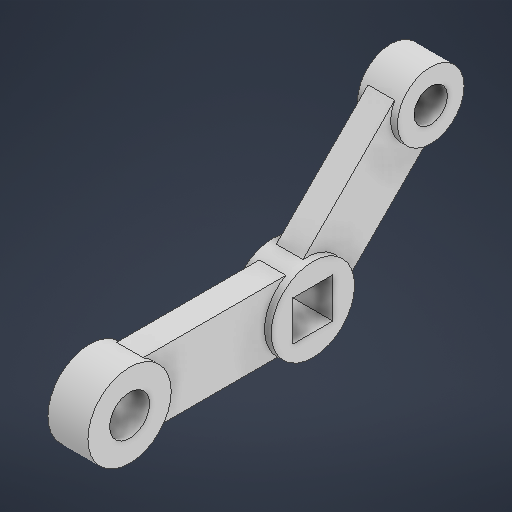
# Autodesk Inventor part: Part4
Saved by Autodesk Inventor 2026 (Build 300175050, 175E)
## iProperties
Created: 2026-04-09
Part Number: Part4
Material: Generic
Document SubType Name: Modeling
Designer: Administrator
Density: 1 g/cm^3
Appearance: Default
Author: Administrator
Autodesk Inventor part; units mm, degrees
ref_plane "YZ Plane" through (0, 0, 0) normal (1, 0, 0) x (0, 1, 0)
ref_plane "XZ Plane" through (0, 0, 0) normal (0, 1, 0) x (-1, 0, 0)
ref_plane "XY Plane" through (0, 0, 0) normal (0, 0, 1) x (1, 0, 0)
sketch "Sketch1" plane through (0, 0, 0) normal (1, 0, 0) x (0, 1, 0)
  circle A0 centre (0, 0) radius 12.5
  line L0 (0, 0) -> (0, -55) construction
  circle A1 centre (0, -55) radius 12.5
  line L1 (0, -55) -> (35.3553, -90.3553) construction
  circle A2 centre (35.3553, -90.3553) radius 10
  line L2 (10.9114, -6.0985) -> (10.9114, -48.9015)
  line L3 (-9.0886, -8.5818) -> (-9.0886, -46.4182)
  line L4 (40.0876, -81.5459) -> (12.4612, -54.0158)
  line L5 (0.7049, -67.4801) -> (25.5516, -92.3268)
  dimension "d0" = 25
  dimension "d1" = 55
  dimension "d2" = 25
  dimension "d3" = 50
  dimension "d4" = 20
  dimension "d5" = 20
  dimension "d7" = 45
  dimension "d8" = 0.1
  constraints: 12 end point, 8 point on circle, 3 centre point, 3 coincident, 3 vertical, 1 parallel
  measures "d0" diameter of A0
  measures "d1" distance of L0.start L0.end
  measures "d2" diameter of A1
  measures "d3" distance of L1.start L1.end
  measures "d4" diameter of A2
  measures "d5" distance between parallel lines of L3 L2
  measures "d7" angle of L1 L0
  measures "d8" angle of L5 L4
extrude "Extrusion1" add sketch "Sketch1" along normal mid plane 8
sketch "Sketch2" plane through (4, 0, 0) normal (1, 0, 0) x (0, 0, -1)
  circle A0 centre (0, 0) radius 12.5
  line L0 (0, 0) -> (55, 0) construction
  circle A1 centre (55, 0) radius 12.5
  line L1 (55, 0) -> (90.3553, 35.3553)
  circle A2 centre (90.3553, 35.3553) radius 10
  dimension "d11" = 25
  dimension "d12" = 55
  dimension "d13" = 25
  dimension "d14" = 50
  dimension "d15" = 45
  dimension "d16" = 20
  constraints: 4 end point, 3 centre point, 3 coincident, 1 horizontal
  measures "d11" diameter of A0
  measures "d12" distance of L0.start L0.end
  measures "d13" diameter of A1
  measures "d14" distance of L1.start L1.end
  measures "d15" angle of L0 L1
  measures "d16" diameter of A2
extrude "Extrusion2" add sketch "Sketch2" along normal blind 2
sketch "Sketch3" plane through (-4, 0, 0) normal (-1, 0, 0) x (0, 0, 1)
  line L0 (0, 0) -> (-55, 0) construction
  line L1 (-55, 0) -> (-90.3553, 35.3553) construction
  circle A0 centre (-90.3553, 35.3553) radius 10
  circle A1 centre (-55, 0) radius 12.5
  circle A2 centre (0, 0) radius 12.5
  dimension "d19" = 55
  dimension "d20" = 50
  dimension "d21" = 45
  dimension "d22" = 20
  dimension "d23" = 25
  dimension "d24" = 25
  constraints: 4 end point, 3 centre point, 3 coincident, 1 horizontal
  measures "d19" distance of L0.start L0.end
  measures "d20" distance of L0.end L1.end
  measures "d21" angle of L0 L1
  measures "d22" diameter of A0
  measures "d23" diameter of A1
  measures "d24" diameter of A2
extrude "Extrusion3" add sketch "Sketch3" along normal blind 2
sketch "Sketch4" plane through (6, 0, 0) normal (1, 0, 0) x (0, 0, -1)
  circle A0 centre (0, 0) radius 6
  line L0 (0, 0) -> (55, 0) construction
  line L1 (55, 0) -> (90.3553, 35.3553) construction
  line L2 (49, -6) -> (61, -6)
  line L3 (61, -6) -> (61, 6)
  line L4 (61, 6) -> (49, 6)
  line L5 (49, 6) -> (49, -6)
  line L6 (49, -6) -> (61, 6) construction
  line L7 (61, -6) -> (49, 6) construction
  circle A1 centre (90.3553, 35.3553) radius 5
  dimension "d27" = 12
  dimension "d28" = 55
  dimension "d29" = 50
  dimension "d30" = 45
  dimension "d31" = 12
  dimension "d32" = 12
  dimension "d33" = 10
  constraints: 16 end point, 2 centre point, 2 coincident, 2 horizontal, 2 midpoint, 2 parallel, 1 perpendicular
  measures "d27" diameter of A0
  measures "d28" distance of L0.start L0.end
  measures "d29" distance of L0.end L1.end
  measures "d30" angle of L0 L1
  measures "d31" distance of L4.end L3.end
  measures "d32" distance of L3.end L2.end
  measures "d33" diameter of A1
extrude "Extrusion4" cut sketch "Sketch4" against normal through all
body "Solid1"
